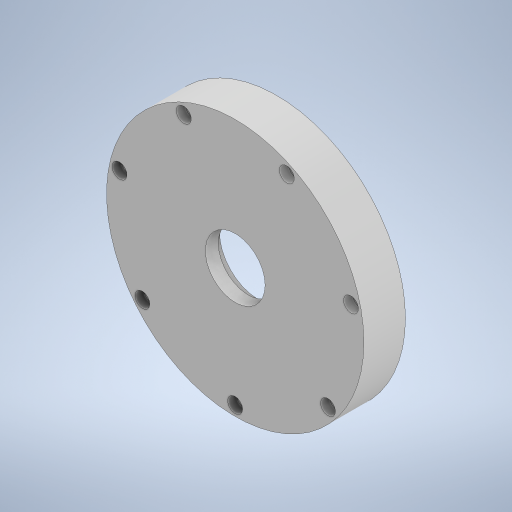
# Autodesk Inventor part: Lid Case
Saved by Autodesk Inventor 2023 (Build 270158000, 158)
## iProperties
Created: 2023-01-18
Part Number: Lid Case
Material: Generic
Document SubType Name: Modeling
Designer: caden
Density: 1 g/cm^3
Appearance: Default
Description: 3D Print
Author: caden
Autodesk Inventor part; units mm, degrees
ref_plane "YZ Plane" through (0, 0, 0) normal (1, 0, 0) x (0, 1, 0)
ref_plane "XZ Plane" through (0, 0, 0) normal (0, 1, 0) x (-1, 0, 0)
ref_plane "XY Plane" through (0, 0, 0) normal (0, 0, 1) x (1, 0, 0)
sketch "Sketch1" plane through (0, 0, 0) normal (0, 0, 1) x (1, 0, 0)
  circle A0 centre (0, 0) radius 77.5
  dimension "d0" = 155
  constraints: 1 centre point, 1 coincident
  measures "d0" diameter of A0
extrude "Extrusion1" add sketch "Sketch1" along normal blind 25
sketch "Sketch2" plane through (0, 0, 0) normal (0, 0, -1) x (-1, 0, 0)
  circle A0 centre (-60, 0) radius 3
  circle A1 centre (0, 0) radius 60 construction
  circle A2 centre (-57.3344, -17.6853) radius 3
  circle A3 centre (-49.5743, -33.7992) radius 3
  circle A4 centre (-37.4094, -46.9099) radius 3
  circle A5 centre (-21.9205, -55.8524) radius 3
  circle A6 centre (-4.4838, -59.8322) radius 3
  circle A7 centre (13.3513, -58.4957) radius 3
  circle A8 centre (30, -51.9615) radius 3
  circle A9 centre (43.9831, -40.8104) radius 3
  circle A10 centre (54.0581, -26.033) radius 3
  circle A11 centre (59.3298, -8.9425) radius 3
  circle A12 centre (59.3298, 8.9425) radius 3
  circle A13 centre (54.0581, 26.033) radius 3
  circle A14 centre (43.9831, 40.8104) radius 3
  circle A15 centre (30, 51.9615) radius 3
  circle A16 centre (13.3513, 58.4957) radius 3
  circle A17 centre (-4.4838, 59.8322) radius 3
  circle A18 centre (-21.9205, 55.8524) radius 3
  circle A19 centre (-37.4094, 46.9099) radius 3
  circle A20 centre (-49.5743, 33.7992) radius 3
  circle A21 centre (-57.3344, 17.6853) radius 3
  dimension "d4" = 120
  dimension "d3" = 6
  dimension "d7" = 360
  constraints: 21 centre point, 1 coincident, 1 horizontal alignment, 45 other
  measures "d3" diameter of A0
extrude "Extrusion2" cut sketch "Sketch2" against normal blind 3
sketch "Sketch3" plane through (0, 0, 25) normal (0, 0, 1) x (1, 0, 0)
  circle A0 centre (0, 0) radius 18
  dimension "d11" = 36
  constraints: 1 centre point, 1 coincident
  measures "d11" diameter of A0
extrude "Extrusion3" cut sketch "Sketch3" against normal through all
sketch "Sketch4" plane through (0, 0, 0) normal (0, 0, -1) x (-1, 0, 0)
  circle A0 centre (0, 0) radius 46
  dimension "d14" = 92
  constraints: 1 centre point, 1 coincident
  measures "d14" diameter of A0
extrude "Extrusion4" cut sketch "Sketch4" against normal blind 11
sketch "Sketch5" plane through (0, 0, 25) normal (0, 0, 1) x (1, 0, 0)
  circle A0 centre (0, 0) radius 71.5 construction
  point P0 (-0.0461, -71.5)
  dimension "d24" = 143
  constraints: 1 coincident, 3 other
hole "Hole" at (-0.0461, -71.5, 25) direction (0, 0, -1) diameter 6 end through all counterbore diameter 9 counterbore depth 5.5
pattern_circular "Circular Pattern1" count 7 over 360 about axis through (0, 0, -10) along (0, 0, 1) of "Hole"
sketch "Sketch6" plane through (0, 0, 0) normal (0, 0, -1) x (-1, 0, 0)
  circle A0 centre (0, 0) radius 65
  dimension "d28" = 130
  constraints: 1 centre point, 1 coincident
  measures "d28" diameter of A0
extrude "Extrusion5" cut sketch "Sketch6" against normal blind 1
sketch "Sketch7" plane through (0, 0, 11) normal (0, 0, -1) x (-1, 0, 0)
  circle A0 centre (0, 0) radius 23.5
  dimension "d31" = 47
  constraints: 1 centre point, 1 coincident
  measures "d31" diameter of A0
extrude "Extrusion6" cut sketch "Sketch7" against normal blind 6.2
body "Solid1"
